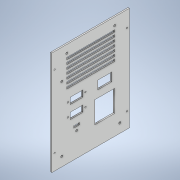
# Autodesk Inventor part: front plate
Saved by Autodesk Inventor 2020.3 (Build 243373000, 373)
## iProperties
Created: 2020-08-09
Part Number: front plate
Material: Generic
Document SubType Name: Modeling
Designer: joesp
Density: 1 g/cm^3
Appearance: Default
Author: joesp
Autodesk Inventor part; units mm, degrees
ref_plane "YZ Plane" through (0, 0, 0) normal (1, 0, 0) x (0, 1, 0)
ref_plane "XZ Plane" through (0, 0, 0) normal (0, 1, 0) x (-1, 0, 0)
ref_plane "XY Plane" through (0, 0, 0) normal (0, 0, 1) x (1, 0, 0)
sketch "Sketch1" plane through (0, 0, 0) normal (1, 0, 0) x (0, 1, 0)
  line L0 (0, 0) -> (147, 0)
  line L1 (147, 0) -> (147, 110)
  line L2 (147, 110) -> (0, 110)
  line L3 (0, 110) -> (0, 0)
  circle A0 centre (124.75, 106.25) radius 1
  circle A1 centre (124.75, 3.75) radius 1
  circle A2 centre (22.25, 3.75) radius 1
  circle A3 centre (22.25, 106.25) radius 1
  dimension "d0" = 102.5
  dimension "d1" = 102.5
  dimension "d2" = 2
  dimension "d3" = 110
  dimension "d4" = 147
  dimension "d5" = 22.25
  dimension "d6" = 22.25
  dimension "d7" = 3.75
  dimension "d8" = 3.75
  constraints: 8 end point, 4 centre point, 3 equal radius, 2 horizontal alignment, 2 parallel, 2 vertical alignment, 1 horizontal, 1 perpendicular
  measures "d0" distance of A1.centre A0.centre
  measures "d1" distance of A3.centre A0.centre
  measures "d2" diameter of A0
  measures "d3" distance of L0.end L1.end
  measures "d4" distance of L1.end L2.end
  measures "d5" distance from line of L1 A0.centre
  measures "d6" distance from line of L3 A3.centre
  measures "d7" distance from line of L2 A0.centre
  measures "d8" distance from line of L0 A1.centre
extrude "Extrusion1" add sketch "Sketch1" along normal blind 2
sketch "Sketch5" plane through (2, 0, 0) normal (1, 0, 0) x (0, 0, -1)
  line L0 (0, 0) -> (0, 147) projected
  line L1 (-110, 147) -> (-110, 0) projected
  circle A0 centre (-13.8284, 13.0004) radius 1.5
  circle A1 centre (-96.1716, 13.0004) radius 1.5
  circle A2 centre (-89, 136.172) radius 1.5
  circle A3 centre (-96.1716, 105.0004) radius 1.5
  circle A4 centre (-21, 136.172) radius 1.5
  line L2 (-110, 0) -> (0, 0) projected
  line L3 (0, 147) -> (-110, 147) projected
  dimension "d94" = 3
  dimension "d116" = 21
  dimension "d117" = 68
  dimension "d118" = 82.3431
  dimension "d119" = 123.1716
  dimension "d120" = 7.1716
  dimension "d121" = 92
  dimension "d122" = 10.828
  constraints: 5 centre point, 4 equal radius, 2 horizontal alignment, 1 vertical alignment
  measures "d94" diameter of A0
  measures "d116" distance from line of L0 A4.centre
  measures "d117" distance of A4.centre A2.centre
  measures "d118" distance of A0.centre A1.centre
  measures "d119" vertical distance of A4.centre A0.centre
  measures "d120" horizontal distance of A4.centre A0.centre
  measures "d121" distance of A3.centre A1.centre
  measures "d122" distance from line of L3 A2.centre
extrude "Extrusion4" cut sketch "Sketch5" against normal through all contours A0 | A1 | A2 | A3 | A4
sketch "Sketch7" plane through (0, 0, 0) normal (-1, 0, 0) x (0, 0, 1)
  line L0 (21, 59.172) -> (49, 59.172)
  line L1 (49, 59.172) -> (49, 28.172)
  line L2 (49, 28.172) -> (21, 28.172)
  line L3 (21, 28.172) -> (21, 59.172)
  line L4 (71, 42.172) -> (79, 42.172)
  line L5 (79, 42.172) -> (79, 39.172)
  line L6 (79, 39.172) -> (71, 39.172)
  line L7 (71, 39.172) -> (71, 42.172)
  line L8 (66, 61.172) -> (84, 61.172)
  line L9 (84, 61.172) -> (84, 52.172)
  line L10 (84, 52.172) -> (66, 52.172)
  line L11 (66, 52.172) -> (66, 61.172)
  line L12 (25, 81.172) -> (45, 81.172)
  line L13 (45, 81.172) -> (45, 69.172)
  line L14 (45, 69.172) -> (25, 69.172)
  line L15 (25, 69.172) -> (25, 81.172)
  circle A0 centre (75, 34.172) radius 1.5
  circle A1 centre (62.5, 56.672) radius 1
  circle A2 centre (87.5, 56.672) radius 1
  line L16 (21, 131.172) -> (89, 131.172)
  line L17 (21, 128.172) -> (89, 128.172)
  line L18 (21, 125.172) -> (89, 125.172)
  line L19 (21, 122.172) -> (89, 122.172)
  line L20 (21, 119.172) -> (89, 119.172)
  line L21 (21, 131.172) -> (21, 89.172)
  line L22 (89, 131.172) -> (89, 89.172)
  line L23 (21, 116.172) -> (89, 116.172)
  line L24 (21, 113.172) -> (89, 113.172)
  line L25 (21, 110.172) -> (89, 110.172)
  line L26 (21, 107.172) -> (89, 107.172)
  line L27 (21, 104.172) -> (89, 104.172)
  line L28 (21, 89.172) -> (89, 89.172)
  circle A3 centre (21, 136.172) radius 1.5 construction
  circle A4 centre (21, 136.172) radius 1.5 projected
  circle A5 centre (89, 136.172) radius 1.5 construction
  circle A6 centre (89, 136.172) radius 1.5 projected
  line L29 (110, 147) -> (110, 0) projected
  line L30 (0, 0) -> (0, 147) projected
  line L31 (21, 101.172) -> (89, 101.172)
  line L32 (89, 98.172) -> (21, 98.172)
  line L33 (21, 95.172) -> (89, 95.172)
  line L34 (21, 92.172) -> (89, 92.172)
  line L35 (66, 79.672) -> (84, 79.672)
  line L36 (84, 79.672) -> (84, 70.672)
  line L37 (84, 70.672) -> (66, 70.672)
  line L38 (66, 70.672) -> (66, 79.672)
  circle A7 centre (62.5, 75.172) radius 1
  circle A8 centre (87.5, 75.172) radius 1
  point P0 (35, 69.172)
  point P1 (35, 59.172)
  point P2 (75, 52.172)
  point P3 (75, 42.172)
  point P4 (75, 39.172)
  point P5 (66, 56.672)
  point P6 (84, 56.672)
  point P7 (66, 75.172)
  point P8 (45, 75.172)
  dimension "d105" = 8
  dimension "d106" = 3
  dimension "d107" = 18
  dimension "d108" = 9
  dimension "d109" = 28
  dimension "d110" = 31
  dimension "d111" = 20
  dimension "d112" = 12
  dimension "d123" = 3
  dimension "d124" = 5
  dimension "d125" = 25
  dimension "d126" = 12.5
  dimension "d127" = 2
  dimension "d129" = 3
  dimension "d130" = 3
  dimension "d131" = 3
  dimension "d133" = 3
  dimension "d134" = 3
  dimension "d135" = 3
  dimension "d136" = 3
  dimension "d137" = 3
  dimension "d138" = 3
  dimension "d140" = 5
  dimension "d141" = 40
  dimension "d142" = 35
  dimension "d143" = 35
  dimension "d144" = 10
  dimension "d146" = 10
  dimension "d150" = 3
  dimension "d151" = 3
  dimension "d152" = 3
  dimension "d154" = 3
  dimension "d155" = 3
  dimension "d156" = 8
  dimension "d157" = 28
  constraints: 70 end point, 16 horizontal, 10 parallel, 9 midpoint, 9 vertical alignment, 7 centre point, 5 horizontal alignment, 5 perpendicular, 3 equal radius, 2 coincident, 2 concentric, 1 collinear, 34 other
  measures "d105" distance of L4.start L4.end
  measures "d106" distance of L6.end L4.start
  measures "d107" distance of L8.start L8.end
  measures "d108" distance of L10.end L8.start
  measures "d109" distance of L0.start L0.end
  measures "d110" distance of L2.end L0.start
  measures "d111" distance of L12.start L12.end
  measures "d112" distance of L12.end L13.end
  measures "d123" diameter of A0
  measures "d124" distance from line of L6 A0.centre
  measures "d125" distance of A2.centre A1.centre
  measures "d126" horizontal distance of point (75, 52.172) A1.centre
  measures "d127" diameter of A1
  measures "d129" distance between parallel lines of L16 L17
  measures "d130" distance between parallel lines of L17 L18
  measures "d131" distance between parallel lines of L18 L19
  measures "d133" distance between parallel lines of L19 L20
  measures "d134" distance between parallel lines of L20 L23
  measures "d135" distance between parallel lines of L23 L24
  measures "d136" distance between parallel lines of L24 L25
  measures "d137" distance between parallel lines of L25 L26
  measures "d138" distance between parallel lines of L26 L27
  measures "d140" distance from line of A4.centre L16
  measures "d141" horizontal distance of A0.centre point (35, 59.172)
  measures "d142" distance from line of L29 A0.centre
  measures "d143" distance from line of L30 point (35, 59.172)
  measures "d144" distance between parallel lines of L14 L0
  measures "d146" distance between parallel lines of L10 L4
  measures "d150" distance between parallel lines of L27 L31
  measures "d151" distance between parallel lines of L31 L32
  measures "d152" distance between parallel lines of L32 L33
  measures "d154" distance between parallel lines of L33 L34
  measures "d155" distance between parallel lines of L34 L28
  measures "d156" distance between parallel lines of L28 L12
  measures "d157" distance between parallel lines of L28 L8
extrude "Extrusion5" cut sketch "Sketch7" against normal through all contours L0 L1 L2 L3 | L4 L5 L6 L7 | L8 L9 L10 L11 | L12 L13 L14 L15 | A0 | A1 | A2 | L16 L22 L17 L21 | L18 L22 L19 L21 | L20 L22 L23 L21 | L24 L22 L25 L21 | L26 L22 L27 L21 | L31 L22 L32 L21 | L33 L22 L34 L21 | L35 L36 L37 L38 | A7 | A8
equation "\"d1\" = d0"
equation "\"d5\" = d6"
equation "\"d7\" = d8"
body "Solid1"
